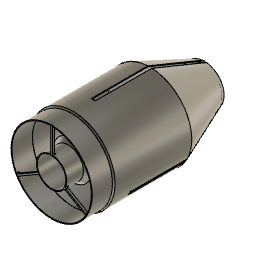
MotorCasingV4 (Autodesk Fusion 360 design; units mm, degrees)
Autodesk Fusion 360 part; units mm, degrees
sketch "Sketch1" plane through (0, 0, 0) normal (0, 0, 1) x (1, 0, 0)
  line L0 (20.1, 0.0308) -> (20.1, 10.0308)
  line L1 (20.1, 10.0308) -> (20.75, 10.6808)
  line L2 (20.75, 10.6808) -> (20.75, 48.6808)
  line L3 (9.1, 75.6808) -> (9.1, 10.6808)
  line L4 (9.1, 0) -> (9.5, 0)
  line L5 (9.5, 10.2808) -> (9.5, 74.2284)
  line L6 (20.35, 48.6025) -> (20.35, 10.8465)
  line L7 (20.35, 10.8465) -> (19.7, 10.1965)
  line L8 (19.7, 10.1965) -> (19.7, 0.0308)
  line L9 (19.7, 0.0308) -> (20.1, 0.0308)
  line L10 (20.35, 48.6025) -> (9.8852, 74.3039)
  line L11 (20.75, 48.6808) -> (9.7565, 75.6808)
  line L12 (9.7565, 75.6808) -> (9.1, 75.6808)
  arc A0 (9.8852, 74.3039) -> (9.5, 74.2284) centre (9.7, 74.2284) ccw
  line L13 (7.1, 0) -> (7.1, 10.6808)
  line L14 (7.1, 0) -> (7.5, 0)
  line L15 (7.5, 0) -> (7.5, 8.2808)
  line L16 (7.5, 8.2808) -> (9.5, 10.2808)
  line L17 (7.1, 10.6808) -> (9.1, 10.6808)
  dimension "d1" = 20.1
  dimension "d2" = 0.4
  dimension "d3" = 0.4
  dimension "d4" = 0.4
  dimension "d5" = 20.75
  dimension "d6" = 135
  dimension "d7" = 9.1
  dimension "d8" = 0.4
  dimension "d10" = 38
  dimension "d11" = 10
  dimension "d14" = 0.2
  dimension "d15" = 2
  dimension "d16" = 2
  dimension "d17" = 0.4
  dimension "d18" = 65
  dimension "d19" = 27
  dimension "d20" = 0.4
  dimension "d21" = 135
  constraint vertical L0
  constraint parallel L0 L2
  constraint parallel L0 L3
  constraint perpendicular L3 L4
  constraint perpendicular L4 L5
  constraint parallel L5 L6
  constraint parallel L5 L8
  constraint perpendicular L0 L9
  constraint parallel L1 L7
  constraint parallel L10 L11
  constraint perpendicular L3 L12
  constraint tangent L10 A0
  constraint tangent L5 A0
  constraint parallel L5 L13
  constraint perpendicular L13 L14
  constraint perpendicular L14 L15
  constraint perpendicular L3 L17
  measures "d1" distance of origin L0
  measures "d2" distance of L0 L8
  measures "d3" distance of L2 L6
  measures "d4" distance of L1 L7
  measures "d5" distance of origin L2
  measures "d6" angle of L0 L1
  measures "d7" distance of origin L3 L0.start
  measures "d8" distance of L3 L5
  measures "d10" distance of L1.end L2.end
  measures "d11" distance of L0.start L0.end
  measures "d14" radius of A0
  measures "d15" distance of L13.end L3.end
  measures "d16" distance of L5 L15
  measures "d17" vertical distance of L5.start L3.end
  measures "d18" distance of L12 L17
  measures "d19" distance of L2.end L12
  measures "d20" distance of L10 L11
  measures "d21" angle of L5 L16
revolve "Revolve1" add sketch "Sketch1" angle 360 about axis through (0, 1.75, 0) along (0, 1, 0)
sketch "Sketch2" plane through (0, 0, 0) normal (0, 1, 0) x (1, 0, 0)
  line L0 (-0.4, -20.096) -> (-0.4, -7.3892)
  line L1 (0.4, -20.096) -> (0.4, -7.3892)
  arc A0 (-0.4, -20.096) -> (0.4, -20.096) centre (0, 0) ccw
  arc A1 (-0.4, -7.3892) -> (0.4, -7.3892) centre (0, 0) ccw
  arc A2 (6.5992, 3.3482) -> (6.1992, 4.041) centre (0, 0) ccw
  line L2 (17.6037, 9.7016) -> (6.5992, 3.3482)
  arc A3 (17.6037, 9.7016) -> (17.2037, 10.3944) centre (0, 0) ccw
  line L3 (17.2037, 10.3944) -> (6.1992, 4.041)
  arc A4 (-6.1992, 4.041) -> (-6.5992, 3.3482) centre (0, 0) ccw
  line L4 (-17.2037, 10.3944) -> (-6.1992, 4.041)
  arc A5 (-17.2037, 10.3944) -> (-17.6037, 9.7016) centre (0, 0) ccw
  line L5 (-17.6037, 9.7016) -> (-6.5992, 3.3482)
  dimension "d23" = 14.8
  dimension "d24" = 40.2
  dimension "d25" = 0.8
  dimension "d26" = 0.4
  dimension "d28" = 360
  constraint coincident A0.centre A1.centre
  constraint concentric A0 A1
  constraint vertical L0
  constraint parallel L0 L1
  measures "d23" diameter of A1
  measures "d24" diameter of A0
  measures "d25" distance of L0 L1
  measures "d26" distance of A0.centre L0
extrude "Extrude1" add sketch "Sketch2" along normal blind 1
sketch "Sketch4" plane through (0, 75.6808, 0) normal (0, 1, 0) x (-1, 0, 0)
  circle A0 centre (0, 0) radius 9.1
  circle A1 centre (0, 0) radius 9.7565
  line L0 (-1, 9.7051) -> (-1, 25.9808)
  line L1 (1, 9.7051) -> (1, 25.9808)
  arc A2 (1, 25.9808) -> (-1, 25.9808) centre (0, 0) ccw
  arc A3 (1, 9.7051) -> (-1, 9.7051) centre (0, 0) ccw
  line L2 (-8.9049, -3.9865) -> (-23, -12.1244)
  arc A4 (-23, -12.1244) -> (-22, -13.8564) centre (0, 0) ccw
  arc A5 (-8.9049, -3.9865) -> (-7.9049, -5.7186) centre (0, 0) ccw
  line L3 (-7.9049, -5.7186) -> (-22, -13.8564)
  line L4 (7.9049, -5.7186) -> (22, -13.8564)
  arc A6 (22, -13.8564) -> (23, -12.1244) centre (0, 0) ccw
  arc A7 (7.9049, -5.7186) -> (8.9049, -3.9865) centre (0, 0) ccw
  line L5 (8.9049, -3.9865) -> (23, -12.1244)
  dimension "d35" = 2
  dimension "d36" = 1
  dimension "d38" = 360
  constraint concentric A0 A3
  constraint coincident A0.centre A1.centre
  constraint vertical L0
  constraint parallel L0 L1
  measures "d35" distance of L0 L1
  measures "d36" distance of A0.centre L0
extrude "Extrude2" cut sketch "Sketch4" against normal blind 55 contours A1 L0 L1 A2 A3 | A1 L4 A6 A7 L5 | A1 L2 A4 A5 L3
fillet "Fillet1" radius 0.4 3 edges at (0.4, 0.5, 7.4893) (0, 1, 7.5) (-0.4, 0.5, 7.4893)
fillet "Fillet1" radius 0.4 3 edges at (0.4, 0.5154, 19.6959) (-0.4, 0.5154, 19.6959) (0, 1, 19.7)
fillet "Fillet1" radius 0.4 12 edges at (-17.2572, 0.5154, -9.5016) (-17.0607, 1, -9.85) (-16.8572, 0.5154, -10.1944) (-6.6859, 0.5, -3.3983) (-6.4952, 1, -3.75) (-6.2859, 0.5, -4.0911) (17.2572, 0.5154, -9.5016) (17.0607, 1, -9.85) (16.8572, 0.5154, -10.1944) (6.6859, 0.5, -3.3983) (6.4952, 1, -3.75) (6.2859, 0.5, -4.0911)
equation "d1 = ( 40.2 / 2 ) * 1 mm"
equation "d5 = ( 41.5 / 2 ) * 1 mm"
